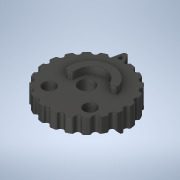
# Autodesk Inventor part: Knob
Saved by Autodesk Inventor 2020.1 (Build 241239000, 239)
## iProperties
Created: 2019-07-16
Part Number: Knob
Material: Generic
Document SubType Name: Modeling
Designer: Petar
Density: 1 g/cm^3
Appearance: Black Only
Mass: 5.28802 g
Surface Area: 31.3053 cm^2
Volume: 5.28802 cm^3
Author: Petar
Autodesk Inventor part; units mm, degrees
ref_plane "YZ Plane" through (0, 0, 0) normal (1, 0, 0) x (0, 1, 0)
ref_plane "XZ Plane" through (0, 0, 0) normal (0, 1, 0) x (-1, 0, 0)
ref_plane "XY Plane" through (0, 0, 0) normal (0, 0, 1) x (1, 0, 0)
sketch "Sketch1" plane through (0, 0, 0) normal (0, 1, 0) x (-1, 0, 0)
  circle A0 centre (0, 0) radius 15.5 construction
  arc A1 (1.2491, -16.7034) -> (-1.2491, -16.7034) centre (0, -16.75) ccw
  arc A2 (6.3496, -15.4998) -> (3.9736, -16.2718) centre (5.176, -15.9302) ccw
  arc A3 (10.8286, -12.7791) -> (8.8074, -14.2475) centre (9.8454, -13.551) ccw
  arc A4 (14.2475, -8.8074) -> (12.7791, -10.8286) centre (13.551, -9.8454) ccw
  arc A5 (16.2718, -3.9736) -> (15.4998, -6.3496) centre (15.9302, -5.176) ccw
  arc A6 (16.7034, 1.2491) -> (16.7034, -1.2491) centre (16.75, 0) ccw
  arc A7 (15.4998, 6.3496) -> (16.2718, 3.9736) centre (15.9302, 5.176) ccw
  arc A8 (12.7791, 10.8286) -> (14.2475, 8.8074) centre (13.551, 9.8454) ccw
  arc A9 (8.8074, 14.2475) -> (10.8286, 12.7791) centre (9.8454, 13.551) ccw
  arc A10 (3.9736, 16.2718) -> (6.3496, 15.4998) centre (5.176, 15.9302) ccw
  arc A11 (-1.2491, 16.7034) -> (1.2491, 16.7034) centre (0, 16.75) ccw
  arc A12 (-6.3496, 15.4998) -> (-3.9736, 16.2718) centre (-5.176, 15.9302) ccw
  arc A13 (-10.8286, 12.7791) -> (-8.8074, 14.2475) centre (-9.8454, 13.551) ccw
  arc A14 (-14.2475, 8.8074) -> (-12.7791, 10.8286) centre (-13.551, 9.8454) ccw
  arc A15 (-16.2718, 3.9736) -> (-15.4998, 6.3496) centre (-15.9302, 5.176) ccw
  arc A16 (-16.7034, -1.2491) -> (-16.7034, 1.2491) centre (-16.75, 0) ccw
  arc A17 (-15.4998, -6.3496) -> (-16.2718, -3.9736) centre (-15.9302, -5.176) ccw
  arc A18 (-12.7791, -10.8286) -> (-14.2475, -8.8074) centre (-13.551, -9.8454) ccw
  arc A19 (-8.8074, -14.2475) -> (-10.8286, -12.7791) centre (-9.8454, -13.551) ccw
  arc A20 (-3.9736, -16.2718) -> (-6.3496, -15.4998) centre (-5.176, -15.9302) ccw
  arc A21 (6.3496, -15.4998) -> (8.8074, -14.2475) centre (0, 0) ccw
  arc A22 (1.2491, -16.7034) -> (3.9736, -16.2718) centre (0, 0) ccw
  arc A23 (-3.9736, -16.2718) -> (-1.2491, -16.7034) centre (0, 0) ccw
  arc A24 (-8.8074, -14.2475) -> (-6.3496, -15.4998) centre (0, 0) ccw
  arc A25 (-12.7791, -10.8286) -> (-10.8286, -12.7791) centre (0, 0) ccw
  arc A26 (-15.4998, -6.3496) -> (-14.2475, -8.8074) centre (0, 0) ccw
  arc A27 (-16.7034, -1.2491) -> (-16.2718, -3.9736) centre (0, 0) ccw
  arc A28 (-16.2718, 3.9736) -> (-16.7034, 1.2491) centre (0, 0) ccw
  arc A29 (-14.2475, 8.8074) -> (-15.4998, 6.3496) centre (0, 0) ccw
  arc A30 (-10.8286, 12.7791) -> (-12.7791, 10.8286) centre (0, 0) ccw
  arc A31 (-6.3496, 15.4998) -> (-8.8074, 14.2475) centre (0, 0) ccw
  arc A32 (-1.2491, 16.7034) -> (-3.9736, 16.2718) centre (0, 0) ccw
  arc A33 (3.9736, 16.2718) -> (1.2491, 16.7034) centre (0, 0) ccw
  arc A34 (8.8074, 14.2475) -> (6.3496, 15.4998) centre (0, 0) ccw
  arc A35 (12.7791, 10.8286) -> (10.8286, 12.7791) centre (0, 0) ccw
  arc A36 (15.4998, 6.3496) -> (14.2475, 8.8074) centre (0, 0) ccw
  arc A37 (16.7034, 1.2491) -> (16.2718, 3.9736) centre (0, 0) ccw
  arc A38 (16.2718, -3.9736) -> (16.7034, -1.2491) centre (0, 0) ccw
  arc A39 (10.8286, -12.7791) -> (12.7791, -10.8286) centre (0, 0) ccw
  arc A40 (14.2475, -8.8074) -> (15.4998, -6.3496) centre (0, 0) ccw
  line L0 (0, -16.75) -> (0, 0) construction
  dimension "d2" = 31
  dimension "d3" = 360
  dimension "d6" = 1.25
  dimension "d7" = 1.25
  constraints: 80 point on circle, 41 centre point, 2 coincident, 2 end point, 1 tangent, 1 vertical, 81 other
  measures "d2" diameter of A0
  measures "d6" radial gap between concentric circles of A0 A23
  measures "d7" radius of A1
extrude "Extrusion1" add sketch "Sketch1" along normal blind 8
fillet "Fillet1" radius 0.5 40 edges at (-15.4998, 4, -6.3496) (-14.2475, 4, -8.8074) (-12.7791, 4, -10.8286) (-10.8286, 4, -12.7791) (-8.8074, 4, -14.2475) (-6.3496, 4, -15.4998) (-3.9736, 4, -16.2718) (-1.2491, 4, -16.7034) (1.2491, 4, -16.7034) (3.9736, 4, -16.2718) (6.3496, 4, -15.4998) (8.8074, 4, -14.2475) (10.8286, 4, -12.7791) (12.7791, 4, -10.8286) (15.4998, 4, -6.3496) (14.2475, 4, -8.8074) (16.2718, 4, -3.9736) (16.7034, 4, -1.2491) (16.7034, 4, 1.2491) (16.2718, 4, 3.9736) (15.4998, 4, 6.3496) (14.2475, 4, 8.8074) (12.7791, 4, 10.8286) (10.8286, 4, 12.7791) (8.8074, 4, 14.2475) (6.3496, 4, 15.4998) (3.9736, 4, 16.2718) (1.2491, 4, 16.7034) (-1.2491, 4, 16.7034) (-3.9736, 4, 16.2718) (-6.3496, 4, 15.4998) (-8.8074, 4, 14.2475) (-10.8286, 4, 12.7791) (-12.7791, 4, 10.8286) (-14.2475, 4, 8.8074) (-15.4998, 4, 6.3496) (-16.2718, 4, 3.9736) (-16.7034, 4, 1.2491) (-16.7034, 4, -1.2491) (-16.2718, 4, -3.9736)
sketch "Sketch2" plane through (0, 0, 0) normal (0, -1, 0) x (1, 0, 0)
  circle A0 centre (0, 0) radius 3.15
  circle A1 centre (0, 0) radius 6
  arc A2 (0, 13) -> (-12.557, 3.3646) centre (0, 0) ccw construction
  arc A3 (1.2491, -16.7034) -> (3.9736, -16.2718) centre (0, 0) ccw construction
  line L0 (16.1793, 4.3352) -> (12.557, 3.3646)
  line L1 (0, 0) -> (0, 17) construction
  line L2 (-16.1793, 4.3352) -> (-12.557, 3.3646)
  arc A4 (16.1793, 4.3352) -> (-16.1793, 4.3352) centre (0, 0) ccw
  arc A5 (12.557, 3.3646) -> (0, 13) centre (0, 0) ccw construction
  arc A6 (-12.557, 3.3646) -> (12.557, 3.3646) centre (0, 0) ccw
  line L3 (-23.3847, 0) -> (23.3847, 0) construction
  dimension "d10" = 6.3
  dimension "d11" = 12
  dimension "d12" = 7
  dimension "d19" = 15
  constraints: 9 point on circle, 6 centre point, 6 end point, 3 coincident, 3 line through centre, 2 symmetric about line, 1 concentric, 1 point on line, 1 vertical
  measures "d10" diameter of A0
  measures "d11" diameter of A1
  measures "d12" radial gap between concentric circles of A1 A2
  measures "d19" angle of L3 L0
extrude "Extrusion2" cut sketch "Sketch2" against normal blind 2 contours L0 A6 L2 A4
extrude "Extrusion3" cut sketch "Sketch2" against normal through all contours A0
chamfer "Chamfer1" distance 2 angle 45 2 edges at (13.9267, 0, 3.7316) (-13.9267, 0, 3.7316)
sketch "Sketch3" plane through (0, 8, 0) normal (0, 1, 0) x (1, 0, 0)
  circle A0 centre (-7.3604, -8.1746) radius 2.55
  circle A1 centre (8.8095, -7.3921) radius 2.55
  line L0 (0, 0) -> (0, -15.5) construction
  arc A2 (1.1784, -16.3329) -> (-1.1784, -16.3329) centre (0, -16.75) ccw construction
  line L1 (0, 0) -> (8.8095, -7.3921) construction
  line L2 (0, 0) -> (-7.3604, -8.1746) construction
  line L3 (-6.2179, -1.6661) -> (-5.2432, -1.4049)
  arc A3 (9.7829, 3.786) -> (-7.4674, -0.8362) centre (1.4489, 0.3882) ccw
  arc A4 (6.9632, 2.7532) -> (-4.5091, -0.3208) centre (1.4489, 0.3882) ccw
  line L4 (8.141, 2.1814) -> (9.1157, 2.4425)
  arc A5 (-7.4674, -0.8362) -> (-6.2179, -1.6661) centre (-6.4767, -0.7002) ccw
  arc A6 (-5.2432, -1.4049) -> (-4.5091, -0.3208) centre (-5.5021, -0.439) ccw
  arc A7 (6.9632, 2.7532) -> (8.141, 2.1814) centre (7.8822, 3.1473) ccw
  arc A8 (9.1157, 2.4425) -> (9.7829, 3.786) centre (8.8569, 3.4085) ccw
  circle A9 centre (-7.3604, -8.1746) radius 0.75
  circle A10 centre (8.8095, -7.3921) radius 0.75
  line L5 (0, 0) -> (1.4489, 0.3882) construction
  line L6 (1.4489, 0.3882) -> (11.1081, 2.9764) construction
  line L7 (0, 0) -> (-9.6593, -2.5882) construction
  line L8 (-5.2432, -1.4049) -> (-5.2432, -1.4049) construction
  line L9 (8.141, 2.1814) -> (8.141, 2.1814) construction
  dimension "d22" = 5.1
  dimension "d23" = 5.1
  dimension "d25" = 50
  dimension "d26" = 1.5
  dimension "d27" = 9
  dimension "d28" = 6
  dimension "d29" = 42
  dimension "d30" = 11.5
  dimension "d31" = 11
  dimension "d32" = 1
  dimension "d33" = 1.5
  dimension "d34" = 1.5
  dimension "d41" = 55
  dimension "d43" = 180
  dimension "d44" = 0
  constraints: 20 end point, 13 point on circle, 10 centre point, 8 tangent, 3 coincident, 3 equal radius, 3 point on line, 2 collinear, 2 perpendicular, 1 parallel, 1 vertical, 1 other
  measures "d22" diameter of A0
  measures "d23" diameter of A1
  measures "d25" angle of L0 L1
  measures "d26" distance of L0.start A3.centre
  measures "d27" radius of A3
  measures "d28" radius of A4
  measures "d29" angle of L0 L2
  measures "d30" distance of L0.start L1.end
  measures "d31" distance of L0.start L2.end
  measures "d32" radius of A5
  measures "d33" diameter of A9
  measures "d34" diameter of A10
  measures "d41" angle of L1 L5
  measures "d43" angle of L4 L3
  measures "d44" distance between parallel lines of L7 L3
extrude "Extrusion4" add sketch "Sketch3" along normal blind 3 contours A5 A3 A8 L4 A7 A4 A6 L3
extrude "Extrusion5" cut sketch "Sketch3" against normal blind 5 contours A0 | A1
extrude "Extrusion6" cut sketch "Sketch3" against normal through all contours A9 | A10
sketch "Sketch4" plane through (0, 8, 0) normal (0, 1, 0) x (1, 0, 0)
  arc A0 (-6.1678, 15.1694) -> (-3.9265, 15.8976) centre (-5.176, 15.9302) ccw projected
  arc A1 (-1.1784, 16.3329) -> (1.1784, 16.3329) centre (0, 16.75) ccw projected
  line L0 (-3.9097, 18.7344) -> (-4.7898, 14.7414)
  line L1 (-2.0709, 19.0256) -> (0, 15.5)
  arc A2 (-1.1784, 16.3329) -> (-1.7005, 16.6635) centre (-1.6497, 16.166) ccw projected
  arc A3 (-3.5321, 16.3734) -> (-3.9265, 15.8976) centre (-3.4266, 15.8846) ccw projected
  arc A4 (-1.7005, 16.6635) -> (-3.5321, 16.3734) centre (0, 0) ccw projected
  arc A5 (-2.0709, 19.0256) -> (-3.9097, 18.7344) centre (-2.9331, 18.5192) ccw
  line L2 (-2.6203, 16.5438) -> (-2.9331, 18.5192) construction
  line L3 (-3.1525, 17.5239) -> (-3.3956, 16.421)
  line L4 (-3.3956, 16.421) -> (-1.845, 16.6666)
  line L5 (-1.845, 16.6666) -> (-2.417, 17.6404)
  arc A6 (-2.417, 17.6404) -> (-3.1525, 17.5239) centre (-2.7619, 17.4378) ccw
  point P0 (-2.6203, 16.5438)
  dimension "d48" = 1
  dimension "d49" = 3
  dimension "d50" = 0
  dimension "d51" = 0.4
  constraints: 12 end point, 8 point on circle, 4 tangent, 2 centre point, 2 point on line, 1 coincident, 1 equal length, 1 line through centre, 1 parallel, 1 perpendicular, 2 other
  measures "d48" radius of A5
  measures "d50" distance edge to line of A4 L4
  measures "d51" radius of A6
extrude "Extrusion7" add sketch "Sketch4" against normal up to surface (8 mm away)
sketch "Sketch5" plane through (0, 8, 0) normal (0, 1, 0) x (1, 0, 0)
  line L0 (-3.3956, 16.421) -> (-3.1525, 17.5239) projected
  arc A0 (-2.417, 17.6404) -> (-3.1525, 17.5239) centre (-2.7619, 17.4378) ccw projected
  line L1 (-2.417, 17.6404) -> (-1.845, 16.6666) projected
  line L2 (-3.458, 16.1379) -> (-2.5108, 15.8524)
  line L3 (-2.5108, 15.8524) -> (-1.6982, 16.4166)
  line L4 (-2.7619, 17.4378) -> (-2.5108, 15.8524) construction
  line L5 (-1.845, 16.6666) -> (-3.3956, 16.421) construction
  line L6 (-3.3956, 16.421) -> (-3.458, 16.1379)
  line L7 (-1.845, 16.6666) -> (-1.6982, 16.4166)
  point P0 (0, 0)
  dimension "d54" = 0.7
  constraints: 10 end point, 2 collinear, 1 perpendicular, 1 other
  measures "d54" distance from line of L5 L2.end
extrude "Extrusion8" cut sketch "Sketch5" against normal through all
fillet "Fillet2" radius 0.25 3 edges at (-1.6982, 4, -16.4166) (-3.458, 4, -16.1379) (-2.5108, 4, -15.8524)
body "Solid1"
